Autodesk Fusion 360 part; units mm, degrees
note: some values were not read from the file. Chosen so that the rebuilt part matches the saved one: which bodies a step acts on; which face or edge a step refers to. Set by a fixed rule: which sketch regions a step uses.
(part 2 of 2)
extrude "Extrude31" add sketch "Sketch26" along normal blind 10 separate body contours L0 L8 L9 L10 L11 | L0 L10 L11 | L3 L4 L5 L12 L13 L14 | L3 L13 L14 | L15 L16 L17 L18 L19 | L20 L21 L22 makes body 10 at (260.7333, 504.8667, 237.6) makes body 11 at (260.7333, -504.8667, 237.6) makes body 12 at (-260.7333, 504.8667, 237.6) makes body 13 at (-260.7333, -504.8667, 237.6)
chamfer "Chamfer2" distance 165.5 distance2 10 4 edges at (-221.8, -465.7, 247.6) (221.8, 465.7, 247.6) (221.8, -465.7, 247.6) (-221.8, 465.7, 247.6) measured on face at (-260.7333, -504.8667, 247.6) measured on face at (260.7333, 504.8667, 247.6) measured on face at (260.7333, -504.8667, 247.6) measured on face at (-260.7333, 504.8667, 247.6) on bodies 10 11 12 13
sketch "Sketch27" plane through (-339.6, 0, 0) normal (1, 0, 0) x (0, 1, 0)
  circle A0 centre (507.5, 315.6) radius 8.75
  circle A1 centre (-72.5, 315.6) radius 8.75
  circle A2 centre (-507.5, 315.6) radius 8.75
  circle A3 centre (72.5, 315.6) radius 8.75
  circle A4 centre (362.5, 315.6) radius 8.75
  circle A5 centre (-217.5, 315.6) radius 8.75
  circle A6 centre (-362.5, 315.6) radius 8.75
  circle A7 centre (217.5, 315.6) radius 8.75
  line L0 (-584.2, 257.6) -> (584.2, 257.6)
  line L1 (584.2, 257.6) -> (584.2, 355.6)
  line L2 (584.2, 355.6) -> (-584.2, 355.6)
  line L3 (-584.2, 355.6) -> (-584.2, 257.6)
  circle A8 centre (-507.5, 315.6) radius 25
  circle A9 centre (-362.5, 315.6) radius 25
  circle A10 centre (-217.5, 315.6) radius 25
  circle A11 centre (-72.5, 315.6) radius 25
  circle A12 centre (72.5, 315.6) radius 25
  circle A13 centre (217.5, 315.6) radius 25
  circle A14 centre (362.5, 315.6) radius 25
  circle A15 centre (507.5, 315.6) radius 25
  dimension "d234" = 50
  dimension "d235" = 50
  dimension "d236" = 50
  dimension "d237" = 50
  dimension "d238" = 50
  dimension "d239" = 50
  dimension "d240" = 50
  dimension "d241" = 50
  constraint concentric A2 A8
  constraint concentric A6 A9
  constraint concentric A5 A10
  constraint concentric A1 A11
  constraint concentric A3 A12
  constraint concentric A7 A13
  constraint concentric A4 A14
  constraint concentric A0 A15
  measures "d234" diameter of A8
  measures "d235" diameter of A9
  measures "d236" diameter of A10
  measures "d237" diameter of A11
  measures "d238" diameter of A12
  measures "d239" diameter of A13
  measures "d240" diameter of A14
  measures "d241" diameter of A15
extrude "Extrude32" add sketch "Sketch27" along normal blind 1 separate body contours A8 | A9 | A10 | A11 | A12 | A13 | A14 | A15 makes body 14 at (-339.6, 236.9577, 313.9233) makes body 15 at (-339.6, -198.0423, 313.9233) makes body 16 at (-339.6, -343.0423, 313.9233) makes body 17 at (-339.6, 381.9577, 313.9233) makes body 18 at (-339.6, 91.9577, 313.9233) makes body 19 at (-339.6, -518.6809, 331.6125) makes body 20 at (-339.6, -53.0423, 313.9233) makes body 21 at (-339.6, 526.9903, 314.358)
sketch "Sketch28" plane through (339.6, 0, 0) normal (-1, 0, 0) x (0, -1, 0)
  line L0 (-584.2, 257.6) -> (584.2, 257.6)
  line L1 (584.2, 257.6) -> (584.2, 355.6)
  line L2 (584.2, 355.6) -> (-584.2, 355.6)
  line L3 (-584.2, 355.6) -> (-584.2, 257.6)
  circle A0 centre (-217.5, 315.6) radius 8.75
  circle A1 centre (362.5, 315.6) radius 8.75
  circle A2 centre (217.5, 315.6) radius 8.75
  circle A3 centre (-362.5, 315.6) radius 8.75
  circle A4 centre (-72.5, 315.6) radius 8.75
  circle A5 centre (507.5, 315.6) radius 8.75
  circle A6 centre (72.5, 315.6) radius 8.75
  circle A7 centre (-507.5, 315.6) radius 8.75
  circle A8 centre (-507.5, 315.6) radius 25
  circle A9 centre (-362.5, 315.6) radius 25
  circle A10 centre (-217.5, 315.6) radius 25
  circle A11 centre (-72.5, 315.6) radius 25
  circle A12 centre (72.5, 315.6) radius 25
  circle A13 centre (217.5, 315.6) radius 25
  circle A14 centre (362.5, 315.6) radius 25
  circle A15 centre (507.5, 315.6) radius 25
  dimension "d244" = 50
  dimension "d245" = 50
  dimension "d246" = 50
  dimension "d247" = 50
  dimension "d248" = 50
  dimension "d249" = 50
  dimension "d250" = 50
  dimension "d251" = 50
  constraint concentric A7 A8
  constraint concentric A3 A9
  constraint concentric A0 A10
  constraint concentric A4 A11
  constraint concentric A6 A12
  constraint concentric A2 A13
  constraint concentric A1 A14
  constraint concentric A5 A15
  measures "d244" diameter of A8
  measures "d245" diameter of A9
  measures "d246" diameter of A10
  measures "d247" diameter of A11
  measures "d248" diameter of A12
  measures "d249" diameter of A13
  measures "d250" diameter of A14
  measures "d251" diameter of A15
extrude "Extrude33" add sketch "Sketch28" along normal blind 1 separate body contours A8 | A9 | A10 | A11 | A12 | A13 | A14 | A15 makes body 22 at (339.6, -236.9577, 313.9233) makes body 23 at (339.6, 343.0423, 313.9233) makes body 24 at (339.6, 198.0423, 313.9233) makes body 25 at (339.6, -381.9577, 313.9233) makes body 26 at (339.6, -91.9577, 313.9233) makes body 27 at (339.6, 488.0423, 313.9233) makes body 28 at (339.6, 53.0423, 313.9233) makes body 29 at (339.6, -526.9903, 314.358)
sketch "Sketch29" plane through (0, 0, 237.6) normal (0, 0, 1) x (-1, 0, 0)
  line L0 (-130, -458.2) -> (-130, -583.2)
  line L1 (-130, -583.2) -> (-90, -583.2)
  line L2 (-90, -583.2) -> (-90, -673.1)
  line L3 (90, -673.1) -> (90, -583.2)
  line L4 (90, -583.2) -> (130, -583.2)
  line L5 (130, -583.2) -> (130, -458.2)
  line L6 (130, -458.2) -> (-130, -458.2)
  line L7 (90, -673.1) -> (-90, -673.1)
  line L8 (-90, -673.1) -> (-90, -593.2)
  line L9 (-90, -593.2) -> (90, -593.2)
  line L10 (90, -593.2) -> (90, -673.1)
  line L11 (-90, -673.1) -> (90, -673.1)
  dimension "d254" = 10
  constraint horizontal L7
  constraint vertical L8
  constraint horizontal L9
  constraint vertical L10
  constraint coincident L2 L8.end
  constraint coincident L3.start L7.start
  measures "d254" distance of L4 L9
extrude "Extrude34" cut sketch "Sketch29" against normal blind 10 contours L2 L3 L7 L8 L9 L10 L11 bodies 1
sketch "Sketch31" plane through (0, 0, 237.6) normal (0, 0, 1) x (-1, 0, 0)
  line L0 (130, 458.2) -> (130, 583.2)
  line L1 (130, 583.2) -> (90, 583.2)
  line L2 (90, 583.2) -> (90, 673.1)
  line L3 (90, 673.1) -> (-90, 673.1)
  line L4 (-90, 673.1) -> (-90, 583.2)
  line L5 (-90, 583.2) -> (-130, 583.2)
  line L6 (-130, 583.2) -> (-130, 458.2)
  line L7 (-130, 458.2) -> (130, 458.2)
  line L8 (-90, 673.1) -> (90, 673.1)
  line L9 (90, 673.1) -> (90, 593.2)
  line L10 (90, 593.2) -> (-90, 593.2)
  line L11 (-90, 593.2) -> (-90, 673.1)
  dimension "d257" = 10
  constraint horizontal L8
  constraint vertical L9
  constraint horizontal L10
  constraint vertical L11
  constraint coincident L2 L9.end
  constraint coincident L3.end L4.start
  measures "d257" distance of L5 L10
extrude "Extrude35" cut sketch "Sketch31" against normal blind 10 contours L2 L3 L4 L8 L9 L10 L11 bodies 1
equation "d3 = ( 730 / 2 ) * 1 mm"
equation "d4 = 55 in / 2"
equation "d31 = 88.5 cm - 14 in"
equation "d35 = 12 in - 2.5 cm"
equation "d38 = 12 in - 2.5 cm"
